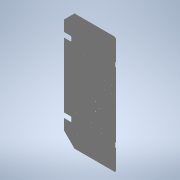
# Autodesk Inventor part: BaseSuperior
Saved by Autodesk Inventor 2022 (Build 260153000, 153)
## iProperties
Created: 2021-10-01
Part Number: BaseSuperior
Material: Steel, Alloy
Document SubType Name: Sheet Metal
Designer: Andres
Density: 7.73 g/cm^3
Sheet Metal Rule: Por defecto_mm
Appearance: Semi-Polished
Author: Andres
Autodesk Inventor part; units mm, degrees
ref_plane "YZ Plane" through (0, 0, 0) normal (1, 0, 0) x (0, 1, 0)
ref_plane "XZ Plane" through (0, 0, 0) normal (0, 1, 0) x (-1, 0, 0)
ref_plane "XY Plane" through (0, 0, 0) normal (0, 0, 1) x (1, 0, 0)
sketch "Sketch1" plane through (0, 0, 0) normal (0, 0, 1) x (1, 0, 0)
  line L0 (0, 20) -> (32, 20) construction
  line L1 (32, 20) -> (32, 206.6274) construction
  line L2 (32, 206.6274) -> (2.6274, 236) construction
  line L3 (2.6274, 236) -> (-370.6274, 236) construction
  line L4 (-370.6274, 236) -> (-480, 126.6274) construction
  line L5 (-480, 126.6274) -> (-480, -726.6274) construction
  line L6 (-480, -726.6274) -> (-370.6274, -836) construction
  line L7 (-370.6274, -836) -> (2.6274, -836) construction
  line L8 (2.6274, -836) -> (32, -806.6274) construction
  line L9 (32, -806.6274) -> (32, -620) construction
  line L10 (32, -620) -> (0, -620) construction
  line L11 (0, -793.3726) -> (0, -620) construction
  line L12 (-10.6274, -804) -> (0, -793.3726) construction
  line L13 (-357.3726, -804) -> (-10.6274, -804) construction
  line L14 (-448, -713.3726) -> (-357.3726, -804) construction
  line L15 (-448, 113.3726) -> (-448, -713.3726) construction
  line L16 (-357.3726, 204) -> (-448, 113.3726) construction
  line L17 (-10.6274, 204) -> (-357.3726, 204) construction
  line L18 (0, 193.3726) -> (-10.6274, 204) construction
  line L19 (0, 20) -> (0, 193.3726) construction
  line L20 (-4, -16) -> (-4, 16) construction
  line L21 (-4, 16) -> (-444, 16) construction
  line L22 (-444, 16) -> (-444, -16) construction
  line L23 (-4, -16) -> (-444, -16) construction
  line L24 (-390.9357, 16) -> (-390.9357, -16) construction
  line L25 (-390.9357, -584) -> (-390.9357, -616) construction
  line L26 (-4, -616) -> (-4, -584) construction
  line L27 (-464, -584) -> (-4, -584) construction
  line L28 (-464, -616) -> (-464, -584) construction
  line L29 (-464, -616) -> (-4, -616) construction
  line L30 (32, -20) -> (0, -20) construction
  line L31 (0, -580) -> (0, -20) construction
  line L32 (0, -580) -> (32, -580) construction
  line L33 (32, -580) -> (32, -20) construction
  line L34 (-357.3726, 204) -> (-10.6274, 204)
  line L35 (33, 21) -> (-5, 21)
  line L36 (-5, 21) -> (-5, -21)
  line L37 (-5, -21) -> (33, -21)
  line L38 (33, -21) -> (33, 21)
  line L39 (33, -579) -> (-5, -579)
  line L40 (-5, -579) -> (-5, -621)
  line L41 (-5, -621) -> (33, -621)
  line L42 (33, -621) -> (33, -579)
  line L43 (-385.8175, 21) -> (-481, 21)
  line L44 (-481, 21) -> (-481, -21)
  line L45 (-481, -21) -> (-385.8175, -21)
  line L46 (-385.8175, -21) -> (-385.8175, 21)
  line L47 (-385.8175, -579) -> (-481, -579)
  line L48 (-481, -579) -> (-481, -621)
  line L49 (-481, -621) -> (-385.8175, -621)
  line L50 (-385.8175, -621) -> (-385.8175, -579)
  line L51 (-10.6274, 204) -> (0, 193.3726)
  line L52 (0, 21) -> (0, 193.3726)
  line L53 (0, -21) -> (0, -579)
  line L54 (0, -621) -> (0, -793.3726)
  line L55 (-10.6274, -804) -> (0, -793.3726)
  line L56 (-357.3726, -804) -> (-448, -713.3726)
  line L57 (-448, -621) -> (-448, -713.3726)
  line L58 (-10.6274, -804) -> (-357.3726, -804)
  line L59 (-448, -579) -> (-448, -21)
  line L60 (-448, 21) -> (-448, 113.3726)
  line L61 (-448, 113.3726) -> (-357.3726, 204)
  line L62 (-471.7703, 20) -> (-464.546, 20) construction
  line L63 (-460.946, -20) -> (-288.146, -20) construction
  line L64 (-386.8175, -16) -> (-386.8175, 16) construction
  line L65 (-471.7703, -580) -> (-464.546, -580) construction
  line L66 (-471.7703, -620) -> (-464.546, -620) construction
  line L67 (-386.8175, -616) -> (-386.8175, -584) construction
  line L68 (-448, 113.3726) -> (0, 113.3726) construction
  line L69 (-448, -713.3726) -> (0, -713.3726) construction
  line L70 (-448, -713.3726) -> (0, 113.3726) construction
  line L71 (-448, 113.3726) -> (0, -713.3726) construction
  line L72 (-224, -300) -> (209.6061, -300) construction
  line L73 (-224, -300) -> (-618.5104, -300) construction
  line L74 (-349, -530.6767) -> (-99, -530.6767) construction
  line L75 (-99, -530.6767) -> (-99, -69.3233) construction
  line L76 (-349, -69.3233) -> (-99, -69.3233) construction
  line L77 (-349, -69.3233) -> (-349, -530.6767) construction
  line L78 (-382.5, -246) -> (-315.5, -246) construction
  line L79 (-315.5, -246) -> (-315.5, -354) construction
  line L80 (-315.5, -354) -> (-382.5, -354) construction
  line L81 (-382.5, -354) -> (-382.5, -246) construction
  line L82 (-382.5, -246) -> (-315.5, -354) construction
  line L83 (-315.5, -246) -> (-382.5, -354) construction
  circle A0 centre (-382.5, -246) radius 1.45
  circle A1 centre (-315.5, -246) radius 1.45
  circle A2 centre (-382.5, -354) radius 1.45
  circle A3 centre (-315.5, -354) radius 1.45
  point P0 (0, 0)
  point P1 (-349, -300)
  point P2 (-349, -300)
  dimension "offset" = 1
  dimension "d1" = 1
  dimension "d2" = 1
  dimension "d3" = 1
  dimension "d4" = 1
  dimension "d5" = 1
  dimension "d6" = 1
  dimension "d7" = 1
  dimension "d10" = 1
  dimension "d15" = 1
  dimension "d18" = 1
  dimension "d19" = 1
  dimension "d20" = 1
  dimension "d21" = 1
  dimension "d22" = 1
  dimension "d24" = 1
  dimension "d38" = 250
  dimension "d39" = 67
  dimension "d40" = 108
  dimension "d41" = 2.9
  dimension "d42" = 2.9
  dimension "d43" = 2.9
  dimension "d44" = 2.9
  measures "offset" distance between parallel lines of L0 L35
  measures "d1" distance between parallel lines of L30 L37
  measures "d2" distance between parallel lines of L20 L36
  measures "d3" distance between parallel lines of L1 L38
  measures "d4" distance between parallel lines of L32 L39
  measures "d5" distance between parallel lines of L33 L42
  measures "d6" distance between parallel lines of L10 L41
  measures "d7" distance between parallel lines of L26 L40
  measures "d10" distance between parallel lines of L5 L44
  measures "d15" distance between parallel lines of L5 L48
  measures "d18" distance between parallel lines of L43 L62
  measures "d19" distance between parallel lines of L46 L64
  measures "d20" distance between parallel lines of L45 L63
  measures "d21" distance between parallel lines of L49 L66
  measures "d22" distance between parallel lines of L67 L50
  measures "d24" distance between parallel lines of L47 L65
  measures "d38" distance of L76.start L75.end
  measures "d39" distance of L78.start L78.end
  measures "d40" distance of L78.end L79.end
  measures "d41" diameter of A0
  measures "d42" diameter of A1
  measures "d43" diameter of A2
  measures "d44" diameter of A3
extrude "Plate1" add sketch "Sketch1" along normal blind 0.5 contours L34 L51 L52 L35 L36 L37 L53 L39 L40 L41 L54 L55 L58 L56 L57 L49 L50 L47 L59 L45 L46 L43 L60 L61 | A0 | A1 | A2 | A3
fillet "Corner Round1" radius 4 8 edges at (-385.8175, 21, 0.25) (-385.8175, -21, 0.25) (-385.8175, -579, 0.25) (-385.8175, -621, 0.25) (-5, -579, 0.25) (-5, -621, 0.25) (-5, -21, 0.25) (-5, 21, 0.25)
sketch "Boceto3" plane through (0, 0, 0.5) normal (0, 0, 1) x (1, 0, 0)
  line L0 (-448, 113.3726) -> (-448, 21) construction
  line L1 (-448, 113.3726) -> (0, 113.3726) construction
  line L2 (-448, -713.3726) -> (-357.3726, -804) construction
  line L3 (0, 113.3726) -> (-448, -713.3726) construction
  line L4 (-448, -621) -> (-448, -713.3726) construction
  line L5 (-448, -713.3726) -> (0, -713.3726) construction
  line L6 (-357.3726, 204) -> (-448, 113.3726) construction
  line L7 (0, -713.3726) -> (-448, 113.3726) construction
  line L8 (-224, -300) -> (173.2728, -300) construction
  line L9 (-224, -300) -> (-609.5128, -300) construction
  line L10 (-349, -530.6767) -> (-99, -530.6767) construction
  line L11 (-99, -530.6767) -> (-99, -69.3233) construction
  line L12 (-99, -69.3233) -> (-349, -69.3233) construction
  line L13 (-349, -69.3233) -> (-349, -530.6767) construction
  line L14 (0, -713.3726) -> (0, 113.3726) construction
  line L15 (0, -793.3726) -> (0, -621) construction
  line L16 (-448, -713.3726) -> (-448, 113.3726) construction
  line L17 (-448, -21) -> (-448, -579) construction
  line L18 (-349, -267) -> (-305, -267) construction
  line L19 (-305, -267) -> (-305, -333) construction
  line L20 (-305, -333) -> (-349, -333) construction
  line L21 (-349, -333) -> (-349, -267) construction
  circle A0 centre (-349, -267) radius 0.8
  circle A1 centre (-305, -267) radius 0.8
  circle A2 centre (-349, -333) radius 0.8
  circle A3 centre (-305, -333) radius 0.8
  line L22 (-349, -486.6767) -> (-283, -486.6767) construction
  line L23 (-283, -486.6767) -> (-283, -530.6767) construction
  line L24 (-283, -530.6767) -> (-349, -530.6767) construction
  line L25 (-349, -530.6767) -> (-349, -486.6767) construction
  line L26 (-349, -69.3233) -> (-283, -69.3233) construction
  line L27 (-283, -69.3233) -> (-283, -113.3233) construction
  line L28 (-283, -113.3233) -> (-349, -113.3233) construction
  line L29 (-349, -113.3233) -> (-349, -69.3233) construction
  line L30 (0, -621) -> (0, -793.3726) construction
  line L31 (-349, -69.3233) -> (-349, -69.3233) construction
  line L32 (-349, -530.6767) -> (-349, -511.6767) construction
  circle A4 centre (-283, -69.3233) radius 0.8
  circle A5 centre (-283, -113.3233) radius 0.8
  circle A6 centre (-349, -113.3233) radius 0.8
  circle A7 centre (-349, -69.3233) radius 0.8
  circle A8 centre (-349, -486.6767) radius 0.8
  circle A9 centre (-349, -530.6767) radius 0.8
  circle A10 centre (-283, -486.6767) radius 0.8
  circle A11 centre (-283, -530.6767) radius 0.8
  line L33 (-179, -530.6767) -> (-179, -69.3233) construction
  line L34 (-58, -530.6767) -> (-58, -69.3233) construction
  line L35 (-305, -333) -> (-349, -267) construction
  line L36 (-349, -333) -> (-305, -267) construction
  circle A12 centre (-179, -435.6767) radius 3
  circle A13 centre (-179, -361.7135) radius 3
  line L37 (-204, -300) -> (-204, -69.3233) construction
  line L38 (-204, -155.0917) -> (-137, -155.0917) construction
  line L39 (-137, -155.0917) -> (-137, -263.0917) construction
  line L40 (-137, -263.0917) -> (-204, -263.0917) construction
  line L41 (-204, -263.0917) -> (-204, -155.0917) construction
  circle A14 centre (-204, -155.0917) radius 1.45
  circle A15 centre (-137, -155.0917) radius 1.45
  circle A16 centre (-204, -263.0917) radius 1.45
  circle A17 centre (-137, -263.0917) radius 1.45
  circle A18 centre (-142.018, -398.695) radius 3
  line L42 (-179, -398.695) -> (-109.8159, -398.695) construction
  line L43 (-214, -713.3726) -> (-214, 113.3726) construction
  line L44 (-448, -579) -> (-389.8175, -579) construction
  line L45 (-448, -579) -> (0, -579) construction
  line L46 (-448, -21) -> (-389.8175, -21) construction
  line L47 (-448, -21) -> (0, -21) construction
  line L48 (-214, -536) -> (-121.7, -536) construction
  line L49 (-121.7, -536) -> (-121.7, -574) construction
  line L50 (-121.7, -574) -> (-214, -574) construction
  line L51 (-214, -574) -> (-214, -536) construction
  circle A19 centre (-214, -536) radius 1.65
  circle A20 centre (-214, -574) radius 1.65
  circle A21 centre (-121.7, -536) radius 1.65
  circle A22 centre (-121.7, -574) radius 1.65
  circle A23 centre (-214, -64) radius 1.65
  circle A24 centre (-214, -26) radius 1.65
  circle A25 centre (-121.7, -64) radius 1.65
  circle A26 centre (-121.7, -26) radius 1.65
  line L52 (-99, -165.3) -> (-39, -165.3) construction
  line L53 (-39, -165.3) -> (-39, -236) construction
  line L54 (-39, -236) -> (-99, -236) construction
  line L55 (-99, -236) -> (-99, -165.3) construction
  circle A27 centre (-99, -165.3) radius 1.5
  circle A28 centre (-39, -165.3) radius 1.5
  circle A29 centre (-39, -236) radius 1.5
  circle A30 centre (-99, -235.6274) radius 1.5
  line L56 (-69, -236) -> (-69, -84.3726) construction
  circle A31 centre (-69, -138) radius 1
  circle A32 centre (-69, -107.1644) radius 1
  line L57 (-448, -713.3726) -> (-448, -621) construction
  line L58 (-461.6137, -692.6226) -> (55.8483, -692.6226) construction
  circle A33 centre (-328, -692.6226) radius 1.5
  circle A34 centre (-241, -692.6226) radius 1.5
  circle A35 centre (-140.7305, -692.6226) radius 1.5
  circle A36 centre (-53.7305, -692.6226) radius 1.5
  circle A37 centre (-328, 92.6226) radius 1.5
  circle A38 centre (-241, 92.6226) radius 1.5
  circle A39 centre (-140.7305, 92.6226) radius 1.5
  circle A40 centre (-53.7305, 92.6226) radius 1.5
  point P0 (0, 0)
  point P1 (-349, -300)
  point P2 (-349, -300)
  point P3 (-349, -69.3233)
  point P4 (-327, -300)
  point P5 (-327, -300)
  point P6 (-349, -69.3233)
  dimension "d45" = 250
  dimension "d46" = 44
  dimension "d47" = 66
  dimension "d48" = 1.6
  dimension "d49" = 1.6
  dimension "d50" = 1.6
  dimension "d51" = 1.6
  dimension "d54" = 66
  dimension "d55" = 44
  dimension "d57" = 19
  dimension "d58" = 44
  dimension "d59" = 66
  dimension "d60" = 1.6
  dimension "d61" = 1.6
  dimension "d62" = 1.6
  dimension "d63" = 1.6
  dimension "d64" = 1.6
  dimension "d65" = 1.6
  dimension "d66" = 1.6
  dimension "d67" = 1.6
  dimension "d68" = 58
  dimension "d69" = 80
  dimension "d71" = 6
  dimension "d72" = 6
  dimension "d73" = 73.9631
  dimension "d74" = 95
  dimension "d75" = 20
  dimension "d76" = 67
  dimension "d77" = 108
  dimension "d78" = 2.9
  dimension "d79" = 2.9
  dimension "d80" = 2.9
  dimension "d81" = 2.9
  dimension "d82" = 6
  dimension "d84" = 36.9815
  dimension "d85" = 36.982
  dimension "d86" = 10
  dimension "d87" = 92.3
  dimension "d88" = 38
  dimension "d89" = 5
  dimension "d90" = 3.3
  dimension "d91" = 3.3
  dimension "d92" = 3.3
  dimension "d93" = 3.3
  dimension "d94" = 60
  dimension "d95" = 70.7
  dimension "d96" = 64
  dimension "d97" = 3
  dimension "d98" = 3
  dimension "d99" = 3
  dimension "d100" = 3
  dimension "d101" = 2
  dimension "d102" = 2
  dimension "d103" = 30.8356
  dimension "d104" = 27.3
  dimension "d105" = 20.75
  dimension "d106" = 3
  dimension "d107" = 3
  dimension "d108" = 3
  dimension "d109" = 3
  dimension "d110" = 87
  dimension "d111" = 87
  dimension "d112" = 100.2695
  dimension "d113" = 120
  constraints: 98 end point, 41 centre point, 29 point on line, 23 coincident, 13 horizontal, 13 parallel, 13 perpendicular, 8 symmetric about line, 5 collinear, 5 midpoint, 2 vertical, 8 other
  measures "d45" distance of L11.end L12.end
  measures "d46" distance of L18.start L18.end
  measures "d47" distance of L18.end L19.end
  measures "d48" diameter of A0
  measures "d49" diameter of A1
  measures "d50" diameter of A2
  measures "d51" diameter of A3
  measures "d54" distance of L22.start L22.end
  measures "d55" distance of L22.end L23.end
  measures "d57" distance of L32.end L10.start
  measures "d58" distance of L26.end L27.end
  measures "d59" distance of L12.end L26.end
  measures "d60" diameter of A4
  measures "d61" diameter of A5
  measures "d62" diameter of A6
  measures "d63" diameter of A7
  measures "d64" diameter of A8
  measures "d65" diameter of A9
  measures "d66" diameter of A10
  measures "d67" diameter of A11
  measures "d68" distance between parallel lines of L14 L34
  measures "d69" distance between parallel lines of L11 L33
  measures "d71" diameter of A12
  measures "d72" diameter of A13
  measures "d73" distance of A12.centre A13.centre
  measures "d74" distance from line of L10 A12.centre
  measures "d75" distance from line of L37 L8.start
  measures "d76" distance of L38.start L38.end
  measures "d77" distance of L38.end L39.end
  measures "d78" diameter of A14
  measures "d79" diameter of A15
  measures "d80" diameter of A16
  measures "d81" diameter of A17
  measures "d82" diameter of A18
  measures "d84" distance from line of L42 A13.centre
  measures "d85" distance from line of A18.centre L33
  measures "d86" distance between parallel lines of L43 L37
  measures "d87" distance of L48.start L48.end
  measures "d88" distance of L48.end L49.end
  measures "d89" distance between parallel lines of L50 L45
  measures "d90" diameter of A19
  measures "d91" diameter of A20
  measures "d92" diameter of A21
  measures "d93" diameter of A22
  measures "d94" distance of L52.start L52.end
  measures "d95" distance of L54.end L52.start
  measures "d96" distance between parallel lines of L8 L54
  measures "d97" diameter of A27
  measures "d98" diameter of A28
  measures "d99" diameter of A29
  measures "d100" diameter of A30
  measures "d101" diameter of A31
  measures "d102" diameter of A32
  measures "d103" distance of A32.centre A31.centre
  measures "d104" distance from line of A31.centre L52
  measures "d105" distance between parallel lines of L5 L58
  measures "d106" diameter of A33
  measures "d107" diameter of A34
  measures "d108" diameter of A35
  measures "d109" diameter of A36
  measures "d110" distance of A34.centre A33.centre
  measures "d111" distance of A36.centre A35.centre
  measures "d112" distance of A35.centre A34.centre
  measures "d113" distance from line of A33.centre L16
extrude "Extrusión1" cut sketch "Boceto3" against normal blind 44
equation "\"d1\" = offset"
equation "\"d2\" = offset"
equation "\"d3\" = offset"
equation "\"d4\" = offset"
equation "\"d5\" = offset"
equation "\"d6\" = offset"
equation "\"d7\" = offset"
equation "\"d10\" = offset"
equation "\"d15\" = offset"
equation "\"d18\" = offset"
equation "\"d19\" = offset"
equation "\"d20\" = offset"
equation "\"d21\" = offset"
equation "\"d22\" = offset"
equation "\"d24\" = offset"
equation "\"d52\" = d58"
equation "\"d16\" = Thickness"
equation "\"BendRadius\" = Thickness"
equation "\"BendReliefWidth\" = Thickness"
equation "\"BendReliefDepth\" = 0.5 * Thickness"
equation "\"CornerReliefSize\" = 4 * Thickness"
equation "\"MinimumRemnant\" = 2 * Thickness"
equation "\"TransitionRadius\" = BendRadius"
equation "\"JacobiRadiusSize\" = BendRadius"
equation "\"GapSize\" = Thickness"
equation "\"Thickness\" = 0.5"
body "Solid1"
